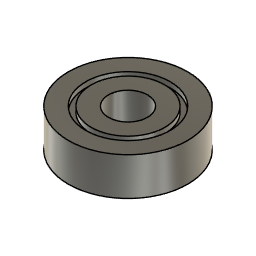
Ruleman (Autodesk Fusion 360 design; units mm, degrees)
Autodesk Fusion 360 part; units mm, degrees
sketch "Boceto1" plane through (0, 0, 0) normal (1, 0, 0) x (0, 1, 0)
  line L0 (5.82, 2.1) -> (8.78, 2.1)
  line L1 (8.78, 2.1) -> (8.78, -2.1)
  line L2 (8.78, -2.1) -> (5.82, -2.1)
  line L3 (5.82, -2.1) -> (5.82, 2.1)
  line L4 (7.3, 2.1) -> (7.3, -2.1) construction
  line L5 (7.8, 2.5) -> (7.8, 3.5)
  line L6 (7.8, 3.5) -> (11, 3.5)
  line L7 (11, 3.5) -> (11, -3.5)
  line L8 (11, -3.5) -> (7.8, -3.5)
  line L9 (7.8, -3.5) -> (7.8, -2.5)
  line L10 (7.8, -2.5) -> (9.18, -2.5)
  line L11 (9.18, -2.5) -> (9.18, 2.5)
  line L12 (9.18, 2.5) -> (7.8, 2.5)
  line L13 (3.6, -3.5) -> (6.8, -3.5)
  line L14 (6.8, -3.5) -> (6.8, -2.5)
  line L15 (6.8, -2.5) -> (5.42, -2.5)
  line L16 (5.42, -2.5) -> (5.42, 2.5)
  line L17 (3.6, 3.5) -> (3.6, -3.5)
  line L18 (6.8, 3.5) -> (3.6, 3.5)
  line L19 (5.42, 2.5) -> (6.8, 2.5)
  line L20 (6.8, 2.5) -> (6.8, 3.5)
  dimension "d1" = 0.4
  dimension "d2" = 0.4
  dimension "d3" = 0.4
  dimension "d4" = 11
  dimension "d5" = 7
  dimension "d6" = 3.5
  dimension "d8" = 0.5
  dimension "d10" = 1
  dimension "d12" = 3.6
  dimension "d13" = 2.96
  constraint horizontal L0
  constraint vertical L1
  constraint horizontal L2
  constraint vertical L3
  constraint midpoint L0 L4.start
  constraint midpoint L2 L4.end
  constraint perpendicular L0 L5
  constraint perpendicular L5 L6
  constraint horizontal L12
  constraint vertical L7
  constraint horizontal L8
  constraint horizontal L10
  constraint vertical L9
  constraint vertical L11
  constraint collinear L5 L9
  constraint equal L5 L9
  constraint symmetric L4 L5.start L19.end
  constraint symmetric L4 L5.end L18.start
  constraint symmetric L4 L6.end L17.start
  constraint symmetric L4 L7.end L13.start
  constraint symmetric L4 L8.end L13.end
  constraint symmetric L4 L9.end L14.end
  constraint symmetric L4 L10.end L15.end
  constraint symmetric L4 L11.end L16.end
  measures "d1" distance of L0 L12
  measures "d2" distance of L2 L10
  measures "d3" distance of L1 L11
  measures "d4" distance of origin L7
  measures "d5" distance of L6.end L7.end
  measures "d6" distance of origin L6
  measures "d8" distance of L4 L5
  measures "d10" distance of L5.start L5.end
  measures "d12" distance of origin L17
  measures "d13" distance of L0.start L0.end
revolve "Revolución1" add sketch "Boceto1" angle 360 about axis through (0, 0, 1.75) along (0, 0, 1) makes body 1 at (0.5397, 5.3931, -0.8333) makes body 2 at (0.8742, 8.7364, 0.7) makes body 3 at (1.0952, 10.9453, -1.1667)
equation "d2 = d1"
equation "d3 = d1"
equation "d6 = d5 / 2"
equation "d13 = 0.4 * ( d4 - d12 )"
